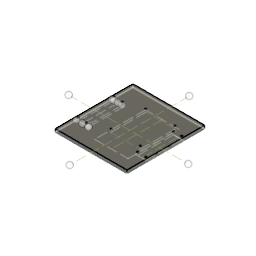
middleChasis (Autodesk Fusion 360 design; units mm, degrees)
part number: 2026-05-17-01-17-44-817
Autodesk Fusion 360 part; units mm, degrees
note: some values were not read from the file. Set by a fixed rule: the direction of a hole.
sketch "Sketch1" plane through (0, 0, 0) normal (0, 0, 1) x (1, 0, 0)
  line L0 (-102.5159, 0.7104) -> (97.4841, 0.7104) construction
  line L1 (0, 100) -> (0, -100) construction
  line L2 (-60, 65.7104) -> (60, 65.7104)
  line L3 (60, 65.7104) -> (60, -64.2896)
  line L4 (60, -64.2896) -> (-60, -64.2896)
  line L5 (-60, -64.2896) -> (-60, 65.7104)
  line L6 (60, 30.7104) -> (39.4499, 30.7104) construction
  line L7 (39.4499, 30.7104) -> (39.4499, -29.2896) construction
  line L8 (39.4499, -29.2896) -> (60, -29.2896) construction
  line L9 (60, -29.2896) -> (60, 30.7104) construction
  line L10 (49.7249, 30.7104) -> (49.7249, -29.2896) construction
  line L11 (56.4749, 30.7104) -> (42.9749, 30.7104) construction
  line L12 (42.9749, 30.7104) -> (42.9749, -29.2896) construction
  line L13 (42.9749, -29.2896) -> (56.4749, -29.2896) construction
  line L14 (56.4749, -29.2896) -> (56.4749, 30.7104) construction
  line L15 (-56.4749, -29.2896) -> (-56.4749, 30.7104) construction
  line L16 (-42.9749, 30.7104) -> (-42.9749, -29.2896) construction
  line L17 (-60, 30.7104) -> (-39.4499, 30.7104) construction
  line L18 (-42.9749, -29.2896) -> (-56.4749, -29.2896) construction
  line L19 (-39.4499, 30.7104) -> (-39.4499, -29.2896) construction
  line L20 (-49.7249, 30.7104) -> (-49.7249, -29.2896) construction
  line L21 (-39.4499, -29.2896) -> (-60, -29.2896) construction
  line L22 (39.4499, 43.2104) -> (-16.5501, 43.2104) construction
  line L23 (-16.5501, 43.2104) -> (-16.5501, -41.7896) construction
  line L24 (-16.5501, -41.7896) -> (39.4499, -41.7896) construction
  line L25 (39.4499, -41.7896) -> (39.4499, 43.2104) construction
  line L26 (35.9499, 40) -> (-13.0501, 40) construction
  line L27 (-13.0501, 40) -> (-13.0501, -18) construction
  line L28 (-13.0501, -18) -> (35.9499, -18) construction
  line L29 (35.9499, -18) -> (35.9499, 40) construction
  line L30 (11.4499, 43.2104) -> (11.4499, -41.7896) construction
  dimension "d1" = 200
  dimension "d2" = 200
  dimension "d3" = 120
  dimension "d4" = 130
  dimension "d5" = 60
  dimension "d6" = 13.5
  dimension "d7" = 56
  dimension "d8" = 85
  dimension "d9" = 49
  dimension "d10" = 58
  constraint perpendicular L0 L1
  constraint horizontal L2
  constraint vertical L3
  constraint horizontal L4
  constraint vertical L5
  constraint symmetric L1 L3 L5
  constraint symmetric L0 L2 L4
  constraint horizontal L6
  constraint vertical L7
  constraint horizontal L8
  constraint vertical L9
  constraint coincident L3 L6.start
  constraint symmetric L0 L6 L8
  constraint midpoint L6 L10.start
  constraint midpoint L8 L10.end
  constraint horizontal L11
  constraint vertical L12
  constraint horizontal L13
  constraint vertical L14
  constraint coincident L6 L11.start
  constraint symmetric L10 L12 L14
  constraint symmetric L1 L6.start L17.start
  constraint symmetric L1 L6.end L17.end
  constraint symmetric L1 L7.end L19.end
  constraint symmetric L1 L10.start L20.start
  constraint symmetric L1 L10.end L20.end
  constraint symmetric L1 L11.start L15.end
  constraint symmetric L1 L11.end L16.start
  constraint symmetric L1 L12.end L16.end
  constraint symmetric L1 L13.end L15.start
  constraint symmetric L1 L8.end L21.end
  constraint horizontal L22
  constraint vertical L23
  constraint horizontal L24
  constraint vertical L25
  constraint symmetric L0 L22 L24
  constraint horizontal L26
  constraint vertical L27
  constraint horizontal L28
  constraint vertical L29
  constraint midpoint L22 L30.start
  constraint midpoint L24 L30.end
  constraint symmetric L27 L29 L30
  measures "d1" distance of L0.start L0.end
  measures "d2" distance of L1.start L1.end
  measures "d3" distance of L2.start L2.end
  measures "d4" distance of L2.start L4.end
  measures "d5" distance of L6.start L8.end
  measures "d6" distance of L11.start L11.end
  measures "d7" distance of L22.start L22.end
  measures "d8" distance of L22.start L24.end
  measures "d9" distance of L26.start L26.end
  measures "d10" distance of L26.start L28.end
extrude "Extrude1" add sketch "Sketch1" along normal blind 5
hole "Hole1" at (56.4749, 30.7104, 0) at (42.9749, 30.7104, 0) at (42.9749, -29.2896, 0) at (56.4749, -29.2896, 0) at (-42.9749, 30.7104, 0) at (-56.4749, 30.7104, 0) at (-56.4749, -29.2896, 0) at (-42.9749, -29.2896, 0) direction (0, 0, 1) diameter 3 depth 5 tip angle 180
hole "Hole2" at (35.9499, 40, 0) at (35.9499, -18, 0) at (-13.0501, 40, 0) at (-13.0501, -18, 0) direction (0, 0, 1) diameter 2.5 depth 5 tip angle 180
